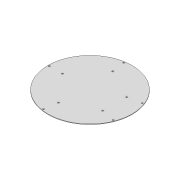
# Autodesk Inventor part: TopandBase
Saved by Autodesk Inventor 2021 (Build 250183000, 183)
## iProperties
Created: 2020-07-30
Part Number: TopandBase
Material: Generic
Document SubType Name: Modeling
Designer: Dan Wikman
Density: 1 g/cm^3
Appearance: Default
Author: Dan Wikman
Autodesk Inventor part; units mm, degrees
ref_plane "YZ Plane" through (0, 0, 0) normal (1, 0, 0) x (0, 1, 0)
ref_plane "XZ Plane" through (0, 0, 0) normal (0, 1, 0) x (-1, 0, 0)
ref_plane "XY Plane" through (0, 0, 0) normal (0, 0, 1) x (1, 0, 0)
sketch "Sketch1" plane through (0, 0, 0) normal (0, 1, 0) x (-1, 0, 0)
  circle A0 centre (-2.1062, 1.0257) radius 576.435
  circle A1 centre (-340.5404, 165.8456) radius 10
  circle A2 centre (-521.3675, 200.9948) radius 10
  line L0 (-296.1915, 1.3356) -> (-698.7298, 1.3356)
  circle A3 centre (-340.5404, -163.1743) radius 10
  circle A4 centre (-521.3675, -198.3235) radius 10
  circle A5 centre (376.435, 0) radius 10
  circle A6 centre (556.435, 0) radius 10
  circle A7 centre (58.8874, 371.8005) radius 10
  circle A8 centre (87.0456, 549.5844) radius 10
  circle A9 centre (58.8874, -371.8005) radius 10
  circle A10 centre (87.0456, -549.5844) radius 10
  point P0 (0, 0)
  point P1 (-578.5411, 1.3356)
  dimension "d34" = 1152.87
  dimension "d52" = 20
  dimension "d55" = 20
  dimension "d58" = 556.435
  dimension "d59" = 20
  dimension "d60" = 376.435
  dimension "d61" = 20
  dimension "d62" = 556.435
  dimension "d65" = 81
  dimension "d69" = 81
  constraints: 10 centre point, 2 end point, 2 symmetric about line, 1 horizontal, 1 point on line, 15 other
  measures "d52" diameter of A1
  measures "d55" diameter of A2
  measures "d58" distance of point (-2.106, 1.026) A2.centre
  measures "d59" diameter of A5
  measures "d60" distance of point (0, 0) A5.centre
  measures "d61" diameter of A6
  measures "d62" distance of point (0, 0) A6.centre
extrude "Extrusion1" add sketch "Sketch1" along normal blind 7
body "Solid1"
